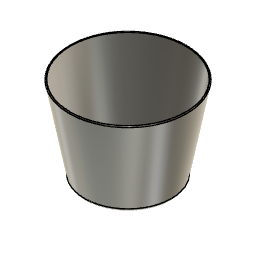
simple flower pot (Autodesk Fusion 360 design; units mm, degrees)
Autodesk Fusion 360 part; units mm, degrees
sketch "top opening geometry for loft" plane through (0, 0, 0) normal (0, 0, 1) x (1, 0, 0)
  circle A0 centre (0, 0) radius 69.85
  dimension "d1" = 139.7
  constraint coincident A0.centre origin
  measures "d1" diameter of A0
ref_plane "WorkPlane1" through (0, 0, -101.6) normal (0, 0, 1) x (1, 0, 0)
sketch "bottom geometry for loft" plane through (0, 0, -101.6) normal (0, 0, 1) x (1, 0, 0)
  circle A0 centre (0, 0) radius 50.8
  dimension "d3" = 101.6
  constraint coincident A0.centre origin
  measures "d3" diameter of A0
loft "Loft1" add profiles "top opening geometry for loft", "bottom geometry for loft" section 1 section 2
shell "Shell1" thickness 1.5 removed faces 1 at (14.777, 14.7334, 0)
sketch "drain hole geometry for circular pattern" plane through (0, 0, -100.1) normal (0, 0, 1) x (-1, 0, 0)
  circle A0 centre (0, 0) radius 49.5551
  circle A1 centre (0, -25) radius 5
  circle A2 centre (23.7764, -7.7254) radius 5
  circle A3 centre (14.6946, 20.2254) radius 5
  circle A4 centre (-14.6946, 20.2254) radius 5
  circle A5 centre (-23.7764, -7.7254) radius 5
  dimension "d5" = 10
  dimension "d7" = 360
  measures "d5" diameter of A1
extrude "Extrude1" cut sketch "drain hole geometry for circular pattern" against normal blind 15 contours A1 | A2 | A3 | A4 | A5
fillet "Fillet1" radius 5 1 edges at (-47.3622, -18.3701, -101.6)
fillet "Fillet2" radius 5 1 edges at (-46.2016, -17.9199, -100.1)
sketch "label location if you want to extrude from object" plane through (0, 0, 0) normal (1, 0, 0) x (0, 1, 0)
  line L0 (35, -50.7175) -> (-37.3016, -50.7175) construction
  line L1 (-37.3016, -50.7175) -> (-37.3016, -30) construction
  line L2 (-37.3016, -30) -> (35, -30) construction
  line L3 (35, -30) -> (35, -50.7175) construction
  dimension "d16" = 15
extrude "Extrude2" [suppressed]
fillet "Fillet3" radius 1 2 edges at (-65.1231, 25.2588, 0) (-63.7002, 24.707, 0)
named bodies: "flower pot"
